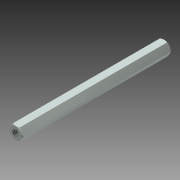
# Autodesk Inventor part: 275-1020
Saved by Autodesk Inventor 2013 (Build 170138000, 138)
## iProperties
Company: Autodesk Inc.
Category: Structure
Part Number: 275-1020
Document SubType Name: Modeling
Designer: Autodesk Inc.
Density: 7.85 g/cm^3
Created: 2012-04-12
Catalog Web Link: http://www.vexrobotics.com/standoffs-8-32.html
Vendor: VEX
Material: Steel
Mass: 19.1268 g
Surface Area: 20.0486 cm^2
Volume: 2.43654 cm^3
Author: Autodesk Inc.
Autodesk Inventor part; units mm, degrees
ref_plane "YZ Plane" through (0, 0, 0) normal (1, 0, 0) x (0, 1, 0)
ref_plane "XZ Plane" through (0, 0, 0) normal (0, 1, 0) x (-1, 0, 0)
sketch "Sketch1" plane through (0, 0, 0) normal (0, 0, 1) x (1, 0, 0)
  line L0 (1.9552, -3.1747) -> (-1.711, -3.1747)
  line L1 (-1.711, -3.1747) -> (-3.5441, 0.0003)
  line L2 (-3.5441, 0.0003) -> (-1.711, 3.1753)
  line L3 (-1.711, 3.1753) -> (1.9552, 3.1753)
  line L4 (1.9552, 3.1753) -> (3.7883, 0.0003)
  line L5 (3.7883, 0.0003) -> (1.9552, -3.1747)
  point P0 (0.1221, 0.0003)
  dimension "d0" = 6.35
  constraints: 12 end point, 1 horizontal, 11 other
  measures "d0" distance between parallel lines of L0 L3
extrude "Extrusion1" add sketch "Sketch1" along normal blind 76.2
ref_plane "Work Plane1" through (-1.711, 0.0003, 0) normal (0, 1, 0) x (1, 0, 0)
sketch "Sketch3" plane through (-1.711, 0.0003, 0) normal (0, 1, 0) x (1, 0, 0)
  line L0 (-1.3251, 0) -> (4.9741, 0)
  line L1 (5.4821, -0.508) -> (5.4821, -75.692)
  line L2 (4.9741, -76.2) -> (-1.3251, -76.2)
  line L3 (-1.8331, -75.692) -> (-1.8331, -0.508)
  line L4 (-1.8331, -0.508) -> (-1.3251, 0)
  line L5 (4.9741, 0) -> (5.4821, -0.508)
  line L6 (-1.3251, -76.2) -> (-1.8331, -75.692)
  line L7 (5.4821, -75.692) -> (4.9741, -76.2)
  line L8 (-1.8331, 0) -> (-1.8331, -76.2) projected
  line L9 (3.6662, 0) -> (5.4993, 0) projected
  line L10 (1.8245, 0) -> (1.8245, -76.2)
  point P0 (-1.8331, 0)
  point P1 (5.4821, -76.2)
  point P2 (5.4821, 0)
  point P3 (-1.8331, -76.2)
  dimension "d5" = 0.508
  dimension "d6" = 0.508
  dimension "d7" = 0.508
  dimension "d8" = 0.508
  dimension "d9" = 0.508
  dimension "d10" = 0.508
  dimension "d11" = 0.508
  dimension "d12" = 0.508
  dimension "d13" = 7.3152
  dimension "d14" = 0
  dimension "d15" = 76.2
  dimension "d16" = 0
  constraints: 18 end point, 8 point on line, 2 midpoint, 2 parallel, 1 horizontal, 1 perpendicular
  measures "d5" distance of L3.end point (-1.833, 0)
  measures "d6" distance of L0.start point (-1.833, 0)
  measures "d7" distance of L0.end point (5.482, 0)
  measures "d8" distance of L1.start point (5.482, 0)
  measures "d9" distance of L2.end point (-1.833, -76.2)
  measures "d10" distance of L3.start point (-1.833, -76.2)
  measures "d11" distance of L1.end point (5.482, -76.2)
  measures "d12" distance of L2.start point (5.482, -76.2)
  measures "d13" distance between parallel lines of L1 L3
  measures "d14" distance between parallel lines of L8 L3
  measures "d15" distance between parallel lines of L0 L2
  measures "d16" distance between parallel lines of L0 L9
revolve "Revolution1" cut sketch "Sketch3" angle 360 about axis through (0.1135, 0.0003, 0) along (0, 0, 1) keep common part contours L0 L5 L1 L7 L2 L10
sketch "Sketch5" plane through (0.1135, 0.0003, 76.2) normal (0, 0, 1) x (1, 0, 0)
  circle A0 centre (0, 0) radius 3.1496 projected
  constraints: 1 coincident
hole "Hole2" at (0.1135, 0.0003, 76.2) at (0.1135, 0.0003, 76.2) direction (0, 0, -1) diameter 3.302 depth 12.7 tip angle 118 thread size "8-32 UNC" class "2B" standard "ANSI Unified Screw Threads"
sketch "Sketch6" plane through (0.1135, 0.0003, 0) normal (0, 0, -1) x (-1, 0, 0)
  circle A0 centre (0, 0) radius 3.1496 projected
  constraints: 1 coincident
hole "Hole3" at (0.1135, 0.0003, 0) direction (0, 0, 1) diameter 3.302 depth 12.7 tip angle 118 thread size "8-32 UNC" class "2B" standard "ANSI Unified Screw Threads"
equation "\"d6\" = d5"
equation "\"d7\" = d5"
equation "\"d8\" = d7"
equation "\"d9\" = d5"
equation "\"d10\" = d9"
equation "\"d11\" = d5"
equation "\"d12\" = d11"
body "Solid1"
